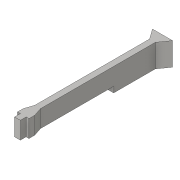
# Autodesk Inventor part: tabwtip_2mm_1128
Saved by Autodesk Inventor 2016 (Build 200138000, 138)
## iProperties
Created: 2017-09-26
Part Number: tabwtip_2mm_1128
Material: Generic
Document SubType Name: Modeling
Designer: Jonathan
Density: 1 g/cm^3
Appearance: Default
Author: Jonathan
Autodesk Inventor part; units mm, degrees
ref_plane "YZ Plane" through (0, 0, 0) normal (1, 0, 0) x (0, 1, 0)
ref_plane "XZ Plane" through (0, 0, 0) normal (0, 1, 0) x (-1, 0, 0)
ref_plane "XY Plane" through (0, 0, 0) normal (0, 0, 1) x (1, 0, 0)
sketch "Sketch1" plane through (0, 0, 0) normal (0, 1, 0) x (-1, 0, 0)
  line L0 (1, 9) -> (-1, 9)
  line L1 (-1, 9) -> (-1, -9)
  line L2 (-1, -9) -> (1, -9)
  line L3 (1, -9) -> (1, 9)
  line L4 (1, 9) -> (-1, -9) construction
  line L5 (-1, 9) -> (1, -9) construction
  line L6 (3.5, -5.5) -> (-3.5, -5.5)
  line L7 (-3.5, -5.5) -> (-3.5, -9)
  line L8 (-3.5, -9) -> (3.5, -9)
  line L9 (3.5, -9) -> (3.5, -5.5)
  line L10 (0, 0) -> (0, -9)
  dimension "d0" = 2
  dimension "d2" = 18
  dimension "d3" = 7
  dimension "d4" = 3.5
  constraints: 22 end point, 4 parallel, 3 midpoint, 3 perpendicular, 2 horizontal, 1 collinear, 1 other
  measures "d0" distance of L2.end L1.end
  measures "d2" distance of L0.end L1.end
  measures "d3" distance of L7.end L8.end
  measures "d4" distance between parallel lines of L8 L6
extrude "Inserted Base" add sketch "Sketch1" along normal blind 8
sketch "Sketch2" plane through (0, 8, 0) normal (0, 1, 0) x (1, 0, 0)
  line L0 (3.5, 5.5) -> (3.5, 9) projected
  line L1 (1, 5.5) -> (3.5, 9)
  line L2 (1, 5.5) -> (3.5, 5.5) projected
  line L3 (3.5, 9) -> (3.5, 5.5)
  line L4 (3.5, 5.5) -> (1, 5.5)
  line L5 (-1, 5.5) -> (-3.5, 9)
  line L6 (-3.5, 9) -> (-3.5, 5.5) projected
  line L7 (-3.5, 9) -> (-3.5, 5.5)
  line L8 (-3.5, 5.5) -> (-1, 5.5) projected
  line L9 (-3.5, 5.5) -> (-1, 5.5)
  point P0 (0, 0)
  constraints: 12 end point, 3 perpendicular, 1 collinear
extrude "Triangle Edges" cut sketch "Sketch2" against normal through all
sketch "Sketch3" plane through (0, 8, 0) normal (0, 1, 0) x (1, 0, 0)
  line L0 (-1, -9) -> (1, -9)
  line L1 (1, -9) -> (1, -41.5)
  line L2 (1, -41.5) -> (-1, -41.5)
  line L3 (-1, -41.5) -> (-1, -9)
  line L4 (1, -9) -> (1, 5.5) projected
  line L5 (-1, -39.5) -> (1, -39.5)
  line L6 (-1, 5.5) -> (-1, -9) projected
  line L7 (1, 5.5) -> (-1, 5.5)
  point P0 (0, 0)
  dimension "d9" = 2
  dimension "d14" = 45
  constraints: 12 end point, 2 horizontal, 2 parallel, 2 perpendicular, 2 point on line, 1 collinear
  measures "d9" distance between parallel lines of L5 L2
  measures "d14" distance between parallel lines of L7 L5
extrude "Tab Extension" add sketch "Sketch3" against normal blind 6 contours L0 L1 L5 L3 | L5 L1 L2 L3
sketch "Sketch4" plane through (0, 8, 0) normal (0, 1, 0) x (1, 0, 0)
  line L0 (2, -39.5) -> (-2, -39.5)
  line L1 (-2, -39.5) -> (-2, -37.5)
  line L2 (-2, -37.5) -> (2, -37.5)
  line L3 (2, -37.5) -> (2, -39.5)
  line L4 (1, -9) -> (1, 5.5) projected
  line L5 (-1, 5.5) -> (-1, -9) projected
  line L6 (1, 5.5) -> (-1, 5.5)
  line L7 (0, 0) -> (0, 5.5)
  line L8 (-1, -41.5) -> (-1, -9) projected
  dimension "d13" = 45
  dimension "d15" = 2
  dimension "d16" = 1
  constraints: 12 end point, 2 horizontal, 2 parallel, 1 midpoint, 1 perpendicular, 1 other
  measures "d13" distance between parallel lines of L6 L0
  measures "d15" distance of L2.end L0.start
  measures "d16" distance between parallel lines of L8 L1
extrude "Electrode rest" add sketch "Sketch4" against normal up to surface (6 mm away)
sketch "Sketch5" plane through (0, 8, 0) normal (0, 1, 0) x (1, 0, 0)
  line L0 (-1, -34.5) -> (1, -34.5)
  line L1 (1, -9) -> (1, -37.5) projected
  line L2 (-2, -37.5) -> (-1, -37.5) projected
  line L3 (-2, -37.5) -> (-1, -37.5)
  line L4 (-1, -34.5) -> (-2, -37.5)
  line L5 (2, -37.5) -> (1, -37.5) projected
  line L6 (1, -37.5) -> (2, -37.5)
  line L7 (2, -37.5) -> (1, -34.5)
  line L8 (-1, -37.5) -> (-1, -34.5)
  line L9 (-1, -37.5) -> (-1, -9) projected
  point P0 (0, 0)
  dimension "d19" = 3
  constraints: 12 end point, 3 horizontal, 1 collinear, 1 point on line
  measures "d19" distance between parallel lines of L0 L2
extrude "Taper" add sketch "Sketch5" against normal up to surface (6 mm away)
body "Solid1"
